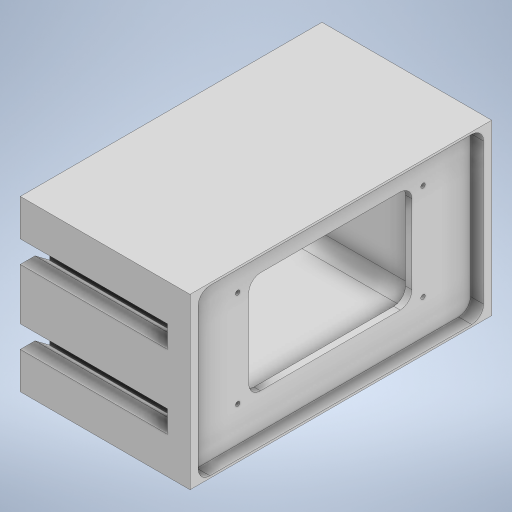
# Autodesk Inventor part: center_fp13
Saved by Autodesk Inventor 2023 (Build 270158000, 158)
## iProperties
Created: 2023-02-13
Part Number: center_fp13
Material: Generic
Document SubType Name: Modeling
Designer: tdal0
Density: 1 g/cm^3
Appearance: Default
Author: tdal0
Autodesk Inventor part; units mm, degrees
ref_plane "YZ Plane" through (0, 0, 0) normal (1, 0, 0) x (0, 1, 0)
ref_plane "XZ Plane" through (0, 0, 0) normal (0, 1, 0) x (-1, 0, 0)
ref_plane "XY Plane" through (0, 0, 0) normal (0, 0, 1) x (1, 0, 0)
sketch "Sketch12" plane through (0, 0, 0) normal (0, 1, 0) x (-1, 0, 0)
  line L0 (0, 0) -> (0, -102.5) construction
  line L1 (0, 0) -> (0, 102.5) construction
  line L2 (0, 102.5) -> (125, 102.5) construction
  line L3 (125, 102.5) -> (125, -102.5) construction
  line L4 (125, -102.5) -> (0, -102.5) construction
  line L5 (0, -102.5) -> (0, 102.5) construction
  line L6 (0, 102.5) -> (45, 102.5) construction
  line L7 (45, 102.5) -> (45, -102.5) construction
  line L8 (45, -102.5) -> (0, -102.5) construction
  line L9 (0, -102.5) -> (0, 102.5) construction
  line L10 (125, 0) -> (125, -217.5) construction
  line L11 (125, 0) -> (125, 217.5) construction
  line L12 (125, 217.5) -> (72.0108, 217.5) construction
  line L13 (45, 217.5) -> (45, 102.5) construction
  line L14 (125, -217.5) -> (72.0108, -217.5) construction
  line L15 (45, -217.5) -> (45, -102.5) construction
  arc A0 (34.5307, 191.4729) -> (34.5307, -191.4729) centre (548.125, 0) ccw construction
  arc A1 (34.5307, -191.4729) -> (72.0108, -217.5) centre (72.0108, -177.5) ccw construction
  arc A2 (72.0108, 217.5) -> (34.5307, 191.4729) centre (72.0108, 177.5) ccw construction
  line L16 (125, -102.5) -> (125, 102.5)
  line L17 (125, 102.5) -> (9.6691, 102.5)
  line L18 (125, -102.5) -> (9.6691, -102.5)
  arc A3 (9.6691, 102.5) -> (9.6691, -102.5) centre (548.125, 0) ccw construction
  line L19 (9.6691, 102.5) -> (9.6691, -102.5)
  dimension "d698" = 102.5
  dimension "d699" = 102.5
  dimension "d700" = 125
  dimension "d701" = 45
  dimension "d702" = 217.5
  dimension "d703" = 217.5
  dimension "d704" = 40
  constraints: 40 end point, 14 point on circle, 6 perpendicular, 6 point on line, 4 centre point, 4 parallel, 4 tangent, 4 vertical, 2 horizontal, 1 collinear, 1 equal radius, 1 midpoint
  measures "d698" distance of L0.start L0.end
  measures "d699" distance of L0.start L1.end
  measures "d700" distance of L3.end L4.end
  measures "d701" distance of L7.end L8.end
  measures "d702" distance of L10.start L10.end
  measures "d703" distance of L10.start L11.end
  measures "d704" radius of A1
extrude "Extrusion12" add sketch "Sketch12" along normal blind 115
sketch "Sketch84" plane through (-125, 0, -102.5) normal (-1, 0, 0) x (0, 0, 1)
  line L0 (33, 107) -> (172, 107)
  line L1 (180, 99) -> (180, 16)
  line L2 (172, 8) -> (33, 8)
  line L3 (25, 16) -> (25, 99)
  line L4 (205, 0) -> (205, 115) projected
  line L5 (0, 0) -> (0, 115) projected
  line L6 (0, 115) -> (205, 115) projected
  line L7 (0, 0) -> (205, 0) projected
  arc A0 (33, 107) -> (25, 99) centre (33, 99) ccw
  arc A1 (180, 99) -> (172, 107) centre (172, 99) ccw
  arc A2 (172, 8) -> (180, 16) centre (172, 16) ccw
  arc A3 (25, 16) -> (33, 8) centre (33, 16) ccw
  point P0 (102.5, 0)
  dimension "d705" = 25
  dimension "d706" = 25
  dimension "d707" = 8
  dimension "d708" = 8
  dimension "d709" = 8
  constraints: 8 end point, 8 point on circle, 8 tangent, 4 centre point, 3 equal radius, 2 parallel, 1 horizontal, 1 perpendicular
  measures "d705" distance between parallel lines of L4 L1
  measures "d706" distance between parallel lines of L5 L3
  measures "d707" distance between parallel lines of L6 L0
  measures "d708" distance between parallel lines of L7 L2
  measures "d709" radius of A0
extrude "Extrusion69" cut sketch "Sketch84" against normal blind 102 contours L0 A1 L1 A2 L2 A3 L3 A0
sketch "Sketch85" plane through (-125, 0, -102.5) normal (-1, 0, 0) x (0, 0, 1)
  line L0 (205, 0) -> (205, 97) projected
  line L1 (205, 25) -> (205, 40)
  line L2 (205, 32.5) -> (185, 32.5) construction
  line L3 (185, 32.5) -> (185, 47.5)
  line L4 (185, 32.5) -> (185, 17.5)
  line L5 (205, 40) -> (195, 40)
  line L6 (195, 40) -> (185, 47.5)
  line L7 (205, 25) -> (195, 25)
  line L8 (195, 25) -> (185, 17.5)
  line L9 (0, 0) -> (205, 0) projected
  line L10 (205, 75) -> (205, 90)
  line L11 (205, 82.5) -> (185, 82.5) construction
  line L12 (185, 82.5) -> (185, 97.5)
  line L13 (185, 82.5) -> (185, 67.5)
  line L14 (205, 75) -> (195, 75)
  line L15 (195, 75) -> (185, 67.5)
  line L16 (205, 90) -> (195, 90)
  line L17 (195, 90) -> (185, 97.5)
  line L18 (0, 115) -> (205, 115) projected
  line L19 (0, 0) -> (0, 115) projected
  line L20 (0, 25) -> (10, 25)
  line L21 (0, 25) -> (10, 25) construction
  line L22 (0, 25) -> (0, 40)
  line L23 (10, 40) -> (0, 40)
  line L24 (0, 32.5) -> (20, 32.5) construction
  line L25 (20, 32.5) -> (20, 47.5)
  line L26 (20, 47.5) -> (10, 40)
  line L27 (20, 32.5) -> (20, 17.5)
  line L28 (20, 17.5) -> (10, 25)
  line L29 (0, 90) -> (10, 90)
  line L30 (0, 90) -> (0, 75)
  line L31 (10, 75) -> (0, 75)
  line L32 (0, 82.5) -> (20, 82.5) construction
  line L33 (20, 82.5) -> (20, 97.5)
  line L34 (20, 97.5) -> (10, 90)
  line L35 (20, 82.5) -> (20, 67.5)
  line L36 (20, 67.5) -> (10, 75)
  point P0 (102.5, 0)
  dimension "d712" = 15
  dimension "d713" = 20
  dimension "d714" = 15
  dimension "d715" = 15
  dimension "d717" = 10
  dimension "d718" = 25
  dimension "d719" = 15
  dimension "d720" = 20
  dimension "d721" = 15
  dimension "d722" = 15
  dimension "d723" = 10
  dimension "d728" = 25
  dimension "d732" = 10
  dimension "d734" = 20
  dimension "d735" = 15
  dimension "d736" = 15
  constraints: 66 end point, 10 point on line, 9 horizontal, 8 perpendicular, 4 midpoint, 2 vertical, 1 collinear, 1 other
  measures "d712" distance of L1.start L1.end
  measures "d713" distance of L2.start L2.end
  measures "d714" distance of L2.end L3.end
  measures "d715" distance of L2.end L4.end
  measures "d717" distance of L1.end L5.end
  measures "d718" distance between parallel lines of L9 L7
  measures "d719" distance of L10.start L10.end
  measures "d720" distance of L11.start L11.end
  measures "d721" distance of L11.end L12.end
  measures "d722" distance of L11.end L13.end
  measures "d723" distance of L10.start L14.end
  measures "d732" distance of L20.start L20.end
  measures "d734" distance of L24.start L24.end
  measures "d735" distance of L24.end L25.end
  measures "d736" distance of L24.end L27.end
extrude "Extrusion70" cut sketch "Sketch85" against normal blind 100
sketch "Sketch86" plane through (-9.6691, 0, 102.5) normal (1, 0, 0) x (0, 0, -1)
  line L0 (0, 90) -> (0, 115) construction
  line L1 (0, 0) -> (205, 0) construction
  line L2 (0, 115) -> (205, 0) construction
  line L3 (0, 115) -> (205, 115) construction
  line L4 (205, 115) -> (0, 0) construction
  line L5 (191.5, 1.5) -> (13.5, 1.5)
  line L6 (5.5, 9.5) -> (5.5, 105.5)
  line L7 (13.5, 113.5) -> (191.5, 113.5)
  line L8 (199.5, 105.5) -> (199.5, 9.5)
  line L9 (199.5, 1.5) -> (5.5, 113.5) construction
  line L10 (5.5, 1.5) -> (199.5, 113.5) construction
  arc A0 (13.5, 113.5) -> (5.5, 105.5) centre (13.5, 105.5) ccw
  arc A1 (199.5, 105.5) -> (191.5, 113.5) centre (191.5, 105.5) ccw
  arc A2 (191.5, 1.5) -> (199.5, 9.5) centre (191.5, 9.5) ccw
  arc A3 (5.5, 9.5) -> (13.5, 1.5) centre (13.5, 9.5) ccw
  point P0 (102.5, 0)
  point P1 (102.5, 57.5)
  dimension "d738" = 194
  dimension "d739" = 112
  dimension "d740" = 8
  constraints: 16 end point, 8 point on circle, 8 point on line, 8 tangent, 4 centre point, 3 equal radius, 3 midpoint, 2 parallel, 1 horizontal, 1 perpendicular
  measures "d738" distance of L9.end L10.end
  measures "d739" distance of L10.start L9.end
  measures "d740" radius of A0
extrude "Extrusion71" cut sketch "Sketch86" against normal blind 8.9
sketch "Sketch90" plane through (-18.5691, 0, 102.5) normal (1, 0, 0) x (0, 0, -1)
  circle A0 centre (41.2486, 90.9267) radius 1.5
  circle A1 centre (167.2486, 25.4267) radius 1.5
  circle A2 centre (41.2486, 25.4267) radius 1.5
  circle A3 centre (167.2486, 90.9267) radius 1.5
  line L0 (198.9986, 106.9003) -> (198.9986, 7.9003)
  line L1 (190.9986, 1.9267) -> (13.9986, 1.9267) construction
  line L2 (5.9986, 9.9267) -> (5.9986, 104.9267) construction
  line L3 (13.9986, 112.9267) -> (190.9986, 112.9267) construction
  line L4 (198.9986, 104.9267) -> (198.9986, 9.9267) construction
  arc A4 (13.9986, 112.9267) -> (5.9986, 104.9267) centre (13.9986, 104.9267) ccw
  arc A5 (198.9986, 104.9267) -> (190.9986, 112.9267) centre (190.9986, 104.9267) ccw
  arc A6 (190.9986, 1.9267) -> (198.9986, 9.9267) centre (190.9986, 9.9267) ccw
  arc A7 (5.9986, 9.9267) -> (13.9986, 1.9267) centre (13.9986, 9.9267) ccw
  line L5 (21.3986, 106.3267) -> (186.7486, 106.3267) construction
  line L6 (186.7486, 106.3267) -> (186.7486, 5.5767) construction
  line L7 (186.7486, 5.5767) -> (21.3986, 5.5767) construction
  line L8 (21.3986, 5.5767) -> (21.3986, 106.3267) construction
  line L9 (33.7486, 94.9267) -> (48.7486, 94.9267) construction
  line L10 (48.7486, 94.9267) -> (48.7486, 86.9267) construction
  line L11 (48.7486, 86.9267) -> (33.7486, 86.9267) construction
  line L12 (33.7486, 86.9267) -> (33.7486, 94.9267) construction
  line L13 (33.7486, 94.9267) -> (48.7486, 86.9267) construction
  line L14 (48.7486, 94.9267) -> (33.7486, 86.9267) construction
  line L15 (33.7486, 29.4267) -> (48.7486, 29.4267) construction
  line L16 (48.7486, 29.4267) -> (48.7486, 21.4267) construction
  line L17 (48.7486, 21.4267) -> (33.7486, 21.4267) construction
  line L18 (33.7486, 21.4267) -> (33.7486, 29.4267) construction
  line L19 (33.7486, 29.4267) -> (48.7486, 21.4267) construction
  line L20 (48.7486, 29.4267) -> (33.7486, 21.4267) construction
  line L21 (159.7486, 29.4267) -> (174.7486, 29.4267) construction
  line L22 (174.7486, 29.4267) -> (174.7486, 21.4267) construction
  line L23 (174.7486, 21.4267) -> (159.7486, 21.4267) construction
  line L24 (159.7486, 21.4267) -> (159.7486, 29.4267) construction
  line L25 (159.7486, 29.4267) -> (174.7486, 21.4267) construction
  line L26 (174.7486, 29.4267) -> (159.7486, 21.4267) construction
  line L27 (159.7486, 94.9267) -> (174.7486, 94.9267) construction
  line L28 (174.7486, 94.9267) -> (174.7486, 86.9267) construction
  line L29 (174.7486, 86.9267) -> (159.7486, 86.9267) construction
  line L30 (159.7486, 86.9267) -> (159.7486, 88.953) construction
  line L31 (159.7486, 94.9267) -> (174.7486, 86.9267) construction
  line L32 (174.7486, 94.9267) -> (159.7486, 86.9267) construction
  line L33 (159.7486, 94.9267) -> (159.7486, 84.9003) construction
  line L34 (56.7486, 94.9267) -> (151.7486, 94.9267)
  line L35 (159.7486, 86.9267) -> (159.7486, 33.4267)
  line L36 (151.7486, 25.4267) -> (56.7486, 25.4267)
  line L37 (48.7486, 33.4267) -> (48.7486, 86.9267)
  arc A8 (56.7486, 94.9267) -> (48.7486, 86.9267) centre (56.7486, 86.9267) ccw
  arc A9 (159.7486, 86.9267) -> (151.7486, 94.9267) centre (151.7486, 86.9267) ccw
  arc A10 (151.7486, 25.4267) -> (159.7486, 33.4267) centre (151.7486, 33.4267) ccw
  arc A11 (48.7486, 33.4267) -> (56.7486, 25.4267) centre (56.7486, 33.4267) ccw
  line L38 (0, 90) -> (0, 115) construction
  line L39 (205, 0) -> (205, 25) construction
  line L40 (0, 115) -> (205, 0) construction
  line L41 (205, 0) -> (205, 115) construction
  line L42 (0, 0) -> (0, 115) construction
  line L43 (0, 0) -> (205, 115) construction
  point P0 (102.5, 0)
  point P1 (5.9986, 112.9267)
  point P2 (5.9986, 1.9267)
  point P3 (198.9986, 112.9267)
  point P4 (159.7486, 25.4267)
  point P5 (102.4986, 57.5003)
  dimension "d840" = 3
  dimension "d841" = 3
  dimension "d842" = 3
  dimension "d843" = 3
  dimension "d844" = 193
  dimension "d845" = 111
  dimension "d846" = 8
  dimension "d847" = 8
  dimension "d848" = 165.35
  dimension "d849" = 100.75
  dimension "d850" = 3.65
  dimension "d851" = 15.4
  dimension "d852" = 15.4
  dimension "d853" = 19.85
  dimension "d854" = 19.85
  dimension "d855" = 15
  dimension "d856" = 8
  dimension "d857" = 15
  dimension "d858" = 15
  dimension "d859" = 8
  dimension "d860" = 19.5
  dimension "d861" = 19.85
  dimension "d862" = 19.5
  dimension "d863" = 19.85
  dimension "d864" = 12.25
  dimension "d865" = 0
  dimension "d866" = 8
  dimension "d868" = 15.4
  dimension "d869" = 6.6
  dimension "d870" = 12.25
  constraints: 80 end point, 16 point on circle, 16 tangent, 14 parallel, 12 centre point, 12 point on line, 9 midpoint, 8 perpendicular, 7 horizontal, 5 equal radius
  measures "d840" diameter of A0
  measures "d841" diameter of A1
  measures "d842" diameter of A2
  measures "d843" diameter of A3
  measures "d844" distance of point (5.999, 112.927) point (198.999, 112.927)
  measures "d845" distance of point (5.999, 1.927) point (5.999, 112.927)
  measures "d846" radius of A4
  measures "d847" radius of A5
  measures "d848" distance of L7.start L7.end
  measures "d849" distance of L5.end L7.start
  measures "d850" distance between parallel lines of L1 L7
  measures "d851" distance from line of L5 A0.centre
  measures "d852" distance from line of L5 A3.centre
  measures "d853" distance from line of L7 A1.centre
  measures "d854" distance from line of L7 A2.centre
  measures "d855" distance of L16.end L17.end
  measures "d856" distance of L16.start L16.end
  measures "d857" distance of L22.end L24.start
  measures "d858" distance of L31.end L30.start
  measures "d859" distance of L27.end L31.end
  measures "d860" distance from line of L6 A3.centre
  measures "d861" distance from line of L8 A0.centre
  measures "d862" distance from line of L6 A1.centre
  measures "d863" distance from line of L8 A2.centre
  measures "d864" distance between parallel lines of L4 L6
  measures "d865" distance between parallel lines of L0 L4
  measures "d866" radius of A8
  measures "d868" distance between parallel lines of L2 L8
  measures "d869" distance between parallel lines of L3 L5
  measures "d870" distance between parallel lines of L0 L6
extrude "Extrusion74" cut sketch "Sketch90" against normal blind 10
body "Solid3"
